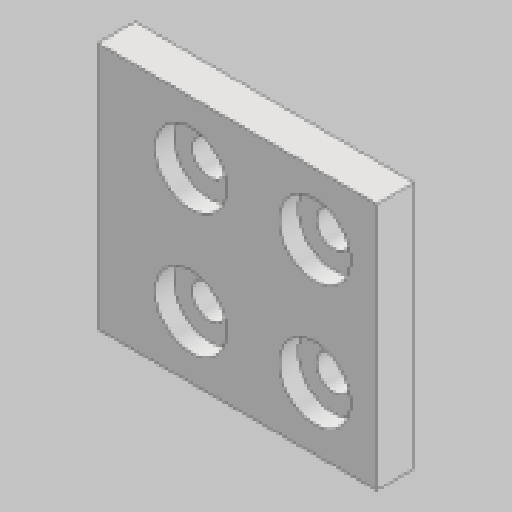
# Autodesk Inventor part: MONTURA LCD
Saved by Autodesk Inventor 2025.4 (Build 294407000, 407)
## iProperties
Created: 2022-05-17
Part Number: MONTURA LCD
Material: Genérico
Document SubType Name: Modeling
Designer: javie
Density: 1 g/cm^3
Appearance: Valor por defecto
Author: javie
Autodesk Inventor part; units mm, degrees
ref_plane "YZ Plane" through (0, 0, 0) normal (1, 0, 0) x (0, 1, 0)
ref_plane "XZ Plane" through (0, 0, 0) normal (0, 1, 0) x (-1, 0, 0)
ref_plane "XY Plane" through (0, 0, 0) normal (0, 0, 1) x (1, 0, 0)
sketch "Boceto1" plane through (0, 0, 0) normal (0, 0, 1) x (1, 0, 0)
  line L0 (29.9998, -9.9999) -> (-15.0002, -9.9999)
  line L1 (-15.0002, -9.9999) -> (-15.0002, 30.0001)
  line L2 (-15.0002, 30.0001) -> (29.9998, 30.0001)
  line L3 (29.9998, 30.0001) -> (29.9998, -9.9999)
  line L4 (-9.8002, -9.9999) -> (-4.883, -9.9999) projected
  line L5 (29.9998, 24.8001) -> (29.9998, 30.0001) projected
  line L6 (-4.8002, 30.0001) -> (-10.0002, 30.0001) projected
  point P0 (0, 0)
  dimension "d0" = 45
  constraints: 8 end point, 3 collinear, 2 parallel, 1 perpendicular, 1 other
  measures "d0" distance of L1.end L2.end
extrude "Extrusión1" add sketch "Boceto1" along normal blind 6
sketch "Boceto8" plane through (0, 0, 6) normal (0, 0, 1) x (1, 0, 0)
  circle A0 centre (19.9998, 0.0001) radius 2.5 projected
  circle A1 centre (19.9998, 20.0001) radius 2.5 projected
  circle A2 centre (-0.0002, 0.0001) radius 2.5 projected
  circle A3 centre (-0.0002, 20.0001) radius 2.5 projected
  circle A4 centre (19.9998, 20.0001) radius 2.75
  circle A5 centre (-0.0002, 20.0001) radius 2.75
  circle A6 centre (-0.0002, 0.0001) radius 2.75
  circle A7 centre (19.9998, 0.0001) radius 2.75
  point P0 (0, 0)
  dimension "d28" = 5.5
  dimension "d29" = 5.5
  dimension "d30" = 5.5
  dimension "d31" = 5.5
  constraints: 4 centre point, 4 coincident
  measures "d28" diameter of A4
  measures "d29" diameter of A5
  measures "d30" diameter of A6
  measures "d31" diameter of A7
extrude "Extrusión8" cut sketch "Boceto8" against normal through all contours A0 | A1 | A2 | A3 | A4 | A5 | A6 | A7
sketch "Boceto9" plane through (0, 0, 6) normal (0, 0, 1) x (1, 0, 0)
  circle A0 centre (19.9998, 0.0001) radius 2.75 projected
  circle A1 centre (-0.0002, 0.0001) radius 2.75 projected
  circle A2 centre (-0.0002, 20.0001) radius 2.75 projected
  circle A3 centre (19.9998, 20.0001) radius 2.75 projected
  circle A4 centre (19.9998, 0.0001) radius 5.75
  circle A5 centre (-0.0002, 0.0001) radius 2.75 projected
  circle A6 centre (-0.0002, 0.0001) radius 5.75
  circle A7 centre (19.9998, 20.0001) radius 2.75 projected
  circle A8 centre (19.9998, 20.0001) radius 5.75
  circle A9 centre (-0.0002, 20.0001) radius 5.75
  point P0 (0, 0)
  dimension "d34" = 11.5
  dimension "d35" = 11.5
  dimension "d36" = 11.5
  dimension "d37" = 11.5
  constraints: 4 centre point, 4 coincident
  measures "d34" diameter of A4
  measures "d35" diameter of A6
  measures "d36" diameter of A8
  measures "d37" diameter of A9
extrude "Extrusión9" cut sketch "Boceto9" against normal blind 3
